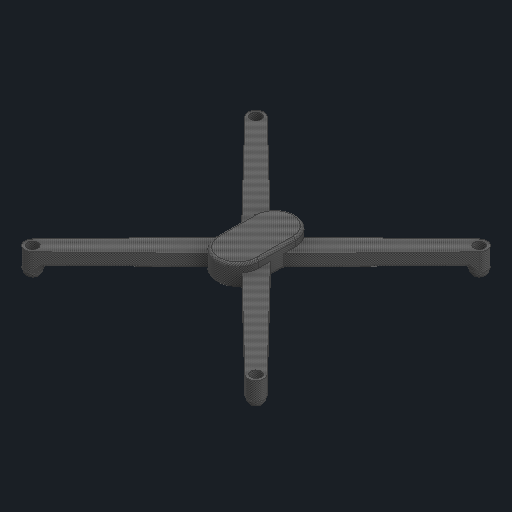
# Autodesk Inventor part: dronek
Saved by Autodesk Inventor 2026 (Build 300175050, 175E)
## iProperties
Created: 2026-03-25
Part Number: dronek
Material: CFRP
Document SubType Name: Modeling
Designer: josef
Mass: 1725.64 g
Surface Area: 1809.9 cm^2
Volume: 1206.74 cm^3
Density: 1.43 g/cm^3
Appearance: Carbon Fiber
Author: josef
Autodesk Inventor part; units mm, degrees
ref_plane "YZ Plane" through (0, 0, 0) normal (1, 0, 0) x (0, 1, 0)
ref_plane "XZ Plane" through (0, 0, 0) normal (0, 1, 0) x (-1, 0, 0)
sketch "Sketch1" plane through (0, 0, 0) normal (0, 1, 0) x (-1, 0, 0)
  circle A0 centre (0, 0) radius 20
  line L0 (0, 0) -> (28.2843, -28.2843)
  line L1 (0, 0) -> (40, 0) construction
  line L2 (0, 0) -> (-113.1371, 113.1371)
  line L3 (0, 0) -> (212.132, 212.132)
  line L4 (0, 0) -> (-113.1371, -113.1371)
  circle A1 centre (212.132, 212.132) radius 15
  circle A2 centre (-212.132, 212.132) radius 15
  circle A3 centre (-212.132, -212.132) radius 15
  circle A4 centre (212.132, -212.132) radius 15
  line L5 (14.1441, 14.1441) -> (222.9139, -201.7037)
  line L6 (-14.1441, -14.1441) -> (201.7037, -222.9139)
  line L7 (-14.1441, 14.1441) -> (201.7037, 222.9139)
  line L8 (14.1441, -14.1441) -> (222.9139, 201.7037)
  line L9 (-14.1441, -14.1441) -> (-222.9139, 201.7037)
  line L10 (14.1441, 14.1441) -> (-201.7037, 222.9139)
  line L11 (14.1441, -14.1441) -> (-201.7037, -222.9139)
  line L12 (-14.1441, 14.1441) -> (-222.9139, -201.7037)
  circle A5 centre (-212.132, -212.132) radius 15
  circle A6 centre (212.132, -212.132) radius 15
  circle A7 centre (212.132, 212.132) radius 15
  circle A8 centre (-212.132, 212.132) radius 15
  circle A9 centre (212.132, -212.132) radius 10
  circle A10 centre (212.132, 212.132) radius 10
  circle A11 centre (-212.132, 212.132) radius 10
  circle A12 centre (-212.132, -212.132) radius 10
  point P0 (14.3759, -13.9045)
  point P1 (14.1441, -14.1441)
  point P2 (13.9045, -14.3759)
  point P3 (13.9045, 14.3759)
  point P4 (14.1441, 14.1441)
  point P5 (14.3759, 13.9045)
  point P6 (-13.9045, -14.3759)
  point P7 (-14.1441, -14.1441)
  point P8 (-14.3759, -13.9045)
  point P9 (-14.3759, 13.9045)
  point P10 (-14.1441, 14.1441)
  point P11 (-13.9045, 14.3759)
  point P12 (27.8244, 0)
  point P13 (222.9139, 201.7037)
  point P14 (201.7037, 222.9139)
  point P15 (0, 27.8244)
  point P16 (-201.7037, 222.9139)
  point P17 (-222.9139, 201.7037)
  point P18 (-27.8244, 0)
  point P19 (-222.9139, -201.7037)
  point P20 (-201.7037, -222.9139)
  point P21 (0, -27.8244)
  dimension "d0" = 40
  dimension "d1" = 40
  dimension "d2" = 45
  dimension "d3" = 160
  dimension "d4" = 300
  dimension "d5" = 160
  dimension "d6" = 90
  dimension "d7" = 90
  dimension "d8" = 90
  dimension "d11" = 30
  dimension "d14" = 360
  dimension "d18" = 360
  dimension "d25" = 30
  dimension "d28" = 360
  dimension "d43" = 20
  dimension "d46" = 360
  constraints: 26 end point, 13 centre point, 6 point on line, 4 coincident, 4 tangent, 2 point on circle, 1 equal length, 1 horizontal, 52 other
  measures "d0" diameter of A0
  measures "d1" distance of L0.start L0.end
  measures "d2" angle of L0 L1
  measures "d3" distance of L0.start L2.end
  measures "d4" distance of L0.start L3.end
  measures "d5" distance of L0.start L4.end
  measures "d6" angle of L0 L4
  measures "d7" angle of L0 L3
  measures "d8" angle of L2 L3
  measures "d11" diameter of A1
  measures "d25" diameter of A5
  measures "d43" diameter of A9
extrude "Extrusion1" add sketch "Sketch1" along normal blind 25 contours A0 L0 L3 | A0 L5 L8 | A0 L3 A1 L8 L5 | L8 L5 A4 L6 L11 A0 | L3 L2 A0 | A0 L10 L7 A1 L3 | A0 L4 L0 | A0 L7 L10 | L4 A0 L2 | A1 | A4 | L11 L6 A0 | A0 L12 L9 A2 L10 L7 | A0 L6 L11 A3 L12 L9 | A2 | A0 L9 L12 | A3 | A9 | A10 | A11 | A12
extrude "Extrusion3" add sketch "Sketch1" against normal blind 25 contours A1 | A4 | A2 | A3 | A9 | A10 | A11 | A12
fillet "Fillet2" radius 8 6 edges at (-201.5254, 0, -201.5254) (-201.5254, 0, 201.5254) (206.5075, 0, 198.2265) (198.3222, 0, 217.9876) (198.3222, 0, -217.9876) (206.5075, 0, -198.2265)
fillet "Fillet3" radius 15 4 edges at (227.132, -25, -212.132) (227.132, -25, 212.132) (-197.132, -25, 212.132) (-197.132, -25, -212.132)
sketch "Sketch3" plane through (0, 25, 0) normal (0, 1, 0) x (1, 0, 0)
  line L0 (-222.9139, 201.7037) -> (-27.8244, 0) projected
  line L1 (-27.8244, 0) -> (-222.9139, -201.7037) projected
  arc A0 (-222.9139, -201.7037) -> (-201.7037, -222.9139) centre (-212.132, -212.132) ccw projected
  line L2 (-201.7037, -222.9139) -> (0, -27.8244) projected
  line L3 (0, -27.8244) -> (201.7037, -222.9139) projected
  arc A1 (201.7037, -222.9139) -> (222.9139, -201.7037) centre (212.132, -212.132) ccw projected
  line L4 (222.9139, -201.7037) -> (27.8244, 0) projected
  line L5 (27.8244, 0) -> (222.9139, 201.7037) projected
  arc A2 (222.9139, 201.7037) -> (201.7037, 222.9139) centre (212.132, 212.132) ccw projected
  line L6 (201.7037, 222.9139) -> (0, 27.8244) projected
  line L7 (0, 27.8244) -> (-201.7037, 222.9139) projected
  arc A3 (-201.7037, 222.9139) -> (-222.9139, 201.7037) centre (-212.132, 212.132) ccw projected
  arc A4 (-210.7923, 189.1711) -> (-189.1711, 210.7923) centre (-212.132, 212.132) ccw projected
  point P0 (0, 0)
sketch "Sketch4" plane through (0, 0, 0) normal (0, -1, 0) x (1, 0, 0)
  circle A0 centre (0, 35) radius 40
  circle A1 centre (0, -35) radius 40
  line L0 (0, 35) -> (0, -75)
  line L1 (40, 35) -> (40, -35)
  line L2 (-40, 35) -> (-40, -35)
  point P0 (0, 0)
  point P1 (0, 0)
  dimension "d36" = 80
  dimension "d37" = 80
  dimension "d38" = 70
  dimension "d39" = 35
  constraints: 6 end point, 5 point on circle, 4 tangent, 2 centre point, 2 point on line, 1 coincident, 1 vertical
  measures "d36" diameter of A0
  measures "d37" diameter of A1
  measures "d38" distance of A1.centre L0.start
  measures "d39" distance of L0.start point (0, 0)
extrude "Extrusion4" add sketch "Sketch4" against normal blind 40
fillet "Fillet4" radius 5 26 edges at (0, 40, 75) (40, 40, 0) (0, 40, -75) (-40, 40, 0) (0, 0, 75) (189.8651, -0.0327, 211.4636) (196.4624, -3.0972, 217.8445) (110.6343, 0, 134.8309) (-195.8525, -2.6341, 217.2546) (-110.6343, 0, 134.8309) (-217.2546, -2.6341, 195.8525) (-125.3962, 0, 100.8797) (-217.0416, -2.4746, -195.6323) (-125.3962, 0, -100.8797) (-195.8525, -2.6341, -217.2546) (-110.6343, 0, -134.8309) (0, 0, -75) (189.8651, -0.0327, -211.4636) (196.4624, -3.0972, -217.8445) (110.6343, 0, -134.8309) (217.2546, -2.6341, -195.8525) (125.3962, 0, -100.8797) (-40, 0, 0) (40, 0, 0) (217.2546, -2.6341, 195.8525) (125.3962, 0, 100.8797)
extrude "Extrusion5" cut sketch "Sketch1" along normal blind 30 contours A9 | A10 | A11 | A12
ref_plane "Work Plane1" through (0, 30, 0) normal (0, 1, 0) x (1, 0, 0)
sketch "Sketch6" plane through (0, 30, 0) normal (0, 1, 0) x (1, 0, 0)
  arc A0 (32.0975, 58.8694) -> (-32.0975, 58.8694) centre (0, 35) ccw projected
  arc A1 (-32.0975, 58.8694) -> (-40, 35) centre (0, 35) ccw projected
  arc A2 (40, 35) -> (-40, 35) centre (0, 35) ccw projected
  arc A3 (40, 35) -> (32.0975, 58.8694) centre (0, 35) ccw projected
  arc A4 (-32.0975, -58.8694) -> (32.0975, -58.8694) centre (0, -35) ccw projected
  arc A5 (32.0975, -58.8694) -> (40, -35) centre (0, -35) ccw projected
  arc A6 (-40, -35) -> (40, -35) centre (0, -35) ccw projected
  arc A7 (-40, -35) -> (-32.0975, -58.8694) centre (0, -35) ccw projected
  line L0 (40, 12.5884) -> (40, -12.5884) projected
  line L1 (40, 35) -> (40, 12.5884) projected
  line L2 (40, -35) -> (40, 35) projected
  line L3 (40, -12.5884) -> (40, -35) projected
  line L4 (-40, -12.5884) -> (-40, 12.5884) projected
  line L5 (-40, -35) -> (-40, -12.5884) projected
  line L6 (-40, 35) -> (-40, -35) projected
  line L7 (-40, 12.5884) -> (-40, 35) projected
  line L8 (25, 50) -> (-25, 50)
  line L9 (-25, 50) -> (-25, -50)
  line L10 (-25, -50) -> (25, -50)
  line L11 (25, -50) -> (25, 50)
  arc A8 (-40, -35) -> (40, -35) centre (0, -35) ccw projected
  point P0 (0, 0)
  point P1 (0, 50)
  point P2 (0, -75)
  dimension "d51" = 50
  dimension "d52" = 100
  dimension "d53" = 15
  dimension "d54" = 25
  constraints: 8 end point, 2 parallel, 1 horizontal, 1 midpoint, 1 perpendicular, 2 other
  measures "d51" distance between parallel lines of L9 L11
  measures "d52" distance from line of L10 point (0, 50)
  measures "d53" distance between parallel lines of L11 L0
  measures "d54" distance from line of point (0, -75) L10
extrude "Extrusion6" cut sketch "Sketch6" against normal blind 20 contours L11 L10 L9 L8
ref_plane "Work Plane2" through (0, 0, -75) normal (0, 0, 1) x (1, 0, 0)
sketch "Sketch7" plane through (0, 0, -75) normal (0, 0, 1) x (1, 0, 0)
  arc A0 (-35, 40) -> (-40, 35) centre (-35, 35) ccw
  line L0 (-35, 40) -> (35, 40)
  arc A1 (40, 35) -> (35, 40) centre (35, 35) ccw
  line L1 (40, 35) -> (-40, 35)
  line L2 (-32.0975, 5) -> (32.0975, 5)
  line L3 (-32.0975, 25) -> (-32.0975, 5)
  line L4 (-40, 25) -> (-32.0975, 25)
  line L5 (-40, 25) -> (-40, 35)
  line L6 (40, 35) -> (-40, 35)
  line L7 (40, 25) -> (40, 35)
  line L8 (32.0975, 25) -> (40, 25)
  line L9 (32.0975, 5) -> (32.0975, 25)
  line L10 (31.1369, 0) -> (-31.1369, 0)
  line L11 (-32.0975, 5) -> (32.0975, 5)
  line L12 (32.0975, 5) -> (186.8158, 5)
  line L13 (32.0975, 5) -> (32.0975, 25)
  line L14 (201.7037, 25) -> (32.0975, 25)
  line L15 (201.7037, -8) -> (201.7037, 25)
  line L16 (32.0975, 5) -> (186.8158, 5)
  ellipse E0 centre (190.2919, 5) end of major axis (190.2919, 0) minor radius 3.4761 (186.8158, 5) -> (190.2919, 0) ccw
  line L17 (190.2919, 0) -> (31.1369, 0)
  line L18 (-186.8158, 5) -> (-32.0975, 5)
  line L19 (-201.7037, -8) -> (-201.7037, 25)
  line L20 (-32.0975, 25) -> (-201.7037, 25)
  line L21 (-32.0975, 25) -> (-32.0975, 5)
  line L22 (-31.1369, 0) -> (-190.2919, 0)
  ellipse E1 centre (-190.2919, 5) end of major axis (-190.2919, 0) minor radius 3.4761 (-190.2919, 0) -> (-186.8158, 5) ccw
  line L23 (-186.8158, 5) -> (-32.0975, 5)
  line L24 (0, 80) -> (0, 0)
  line L25 (118.1245, 20) -> (-40, 20)
  circle A2 centre (0, 20) radius 12.5
  circle A3 centre (0, 20) radius 7.5
  point P0 (0, 40)
extrude "Extrusion7" cut sketch "Sketch7" along normal blind 10 contours A2 L25 A3 L24 | L24 A3 L25 A2 | A3 L25 L24 | L24 L25 A3 | A2 L24 A3 L25 | L25 A3 L24 A2 | L25 A3 L24 | L24 A3 L25
extrude "Extrusion8" cut sketch "Sketch7" along normal blind 20 contours A3 L25 L24 | L24 L25 A3 | L25 A3 L24 | L24 A3 L25
body "Solid1"
